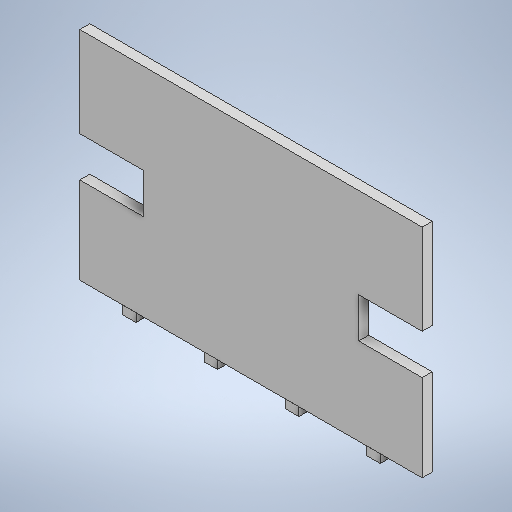
# Autodesk Inventor part: carcasa_piezaFrontal
Saved by Autodesk Inventor 2025.3 (Build 293356030, 356C)
## iProperties
Created: 2025-09-08
Part Number: carcasa_piezaFrontal
Material: Generic
Document SubType Name: Modeling
Designer: brene
Density: 1 g/cm^3
Appearance: Default
Author: brene
Autodesk Inventor part; units mm, degrees
ref_plane "YZ Plane" through (0, 0, 0) normal (1, 0, 0) x (0, 1, 0)
ref_plane "XZ Plane" through (0, 0, 0) normal (0, 1, 0) x (-1, 0, 0)
ref_plane "XY Plane" through (0, 0, 0) normal (0, 0, 1) x (1, 0, 0)
sketch "Sketch1" plane through (0, 0, 0) normal (0, 0, 1) x (1, 0, 0)
  line L0 (0, 0) -> (102.47, 0)
  line L1 (102.47, 0) -> (102.47, 65)
  line L2 (102.47, 65) -> (0, 65)
  line L3 (0, 65) -> (0, 0)
  dimension "d0" = 102.47
  dimension "d1" = 65
  constraints: 8 end point, 2 perpendicular, 1 horizontal, 1 parallel
  measures "d0" distance of L0.start L0.end
  measures "d1" distance of L0.end L1.end
extrude "Extrusion1" add sketch "Sketch1" along normal blind 3
sketch "Sketch2" plane through (0, 0, 3) normal (0, 0, 1) x (1, 0, 0)
  line L0 (0, 0) -> (102.47, 0) projected
  line L1 (51.235, 0) -> (51.235, 65)
  line L2 (102.47, 0) -> (102.47, 26)
  line L3 (102.47, 0) -> (102.47, 65) projected
  line L4 (102.47, 26) -> (83.47, 26)
  line L5 (83.47, 26) -> (83.47, 38)
  line L6 (83.47, 38) -> (102.47, 38)
  line L7 (0, 0) -> (0, 26)
  line L8 (0, 26) -> (19, 26)
  line L9 (19, 26) -> (19, 38)
  line L10 (19, 38) -> (0, 38)
  line L11 (0, 26) -> (0, 38)
  line L12 (0, 65) -> (0, 0) projected
  dimension "d8" = 26
  dimension "d9" = 19
  dimension "d10" = 12
  dimension "d11" = 19
  constraints: 20 end point, 4 symmetric about line, 2 perpendicular, 2 point on line, 1 collinear, 1 midpoint, 1 vertical
  measures "d8" distance of L0.end L2.end
  measures "d9" distance of L2.end L4.end
  measures "d10" distance of L4.end L5.end
  measures "d11" distance of L5.end L6.end
extrude "Extrusion2" cut sketch "Sketch2" against normal blind 50.975
sketch "Sketch3" plane through (0, 0, 0) normal (0, -1, 0) x (1, 0, 0)
  line L0 (0, 0) -> (0, 3) projected
  line L1 (0, 1.5) -> (102.47, 1.5)
  line L2 (102.47, 0) -> (102.47, 3) projected
  line L3 (0, 3) -> (102.47, 3) projected
  line L4 (51.235, 3) -> (51.235, 0)
  line L5 (0, 0) -> (102.47, 0) projected
  line L6 (51.235, 1.5) -> (41.0515, 1.5)
  line L7 (51.235, 1.5) -> (61.4185, 1.5)
  line L8 (41.0515, 1.5) -> (37.0515, 1.5)
  line L9 (39.0515, 1.5) -> (37.0515, 1.5)
  line L10 (37.0515, 1.5) -> (37.0515, 2.85)
  line L11 (41.0515, 1.5) -> (41.0515, 0.15)
  line L12 (37.0515, 2.85) -> (41.0515, 2.85)
  line L13 (41.0515, 2.85) -> (41.0515, 0.15)
  line L14 (41.0515, 0.15) -> (37.0515, 0.15)
  line L15 (37.0515, 0.15) -> (37.0515, 2.85)
  line L16 (65.4185, 1.5) -> (65.4185, 2.85)
  line L17 (65.4185, 2.85) -> (61.4185, 2.85)
  line L18 (61.4185, 2.85) -> (61.4185, 0.15)
  line L19 (61.4185, 0.15) -> (65.4185, 0.15)
  line L20 (65.4185, 0.15) -> (65.4185, 2.85)
  line L21 (37.0515, 1.5) -> (16.6845, 1.5)
  line L22 (26.868, 1.5) -> (26.868, 3)
  line L23 (16.6845, 2.85) -> (12.6845, 2.85)
  line L24 (12.6845, 2.85) -> (12.6845, 0.15)
  line L25 (12.6845, 0.15) -> (16.6845, 0.15)
  line L26 (16.6845, 0.15) -> (16.6845, 2.85)
  line L27 (85.7855, 0.15) -> (85.7855, 2.85)
  line L28 (85.7855, 2.85) -> (89.7855, 2.85)
  line L29 (89.7855, 2.85) -> (89.7855, 0.15)
  line L30 (89.7855, 0.15) -> (85.7855, 0.15)
  dimension "d14" = 10.1835
  dimension "d15" = 10.1835
  dimension "d16" = 4
  dimension "d17" = 2
  dimension "d18" = 1.35
  dimension "d19" = 1.35
  dimension "d20" = 20.367
  constraints: 54 end point, 13 symmetric about line, 7 midpoint, 5 point on line, 3 perpendicular, 2 parallel, 1 collinear, 1 horizontal, 1 vertical
  measures "d14" distance of L6.start L6.end
  measures "d15" distance of L6.start L7.end
  measures "d16" distance of L6.end L8.end
  measures "d17" distance of L9.start L8.end
  measures "d18" distance of L8.end L10.end
  measures "d19" distance of L6.end L11.end
  measures "d20" distance of L8.end L21.end
extrude "Extrusion3" add sketch "Sketch3" along normal blind 2.7 contours L24 L23 L26 L1 | L1 L26 L25 L24 | L11 L14 L15 L1 | L1 L10 L12 L13 | L18 L17 L16 L1 | L1 L20 L19 L18 | L29 L30 L27 L1 | L1 L27 L28 L29
body "Solid1"
